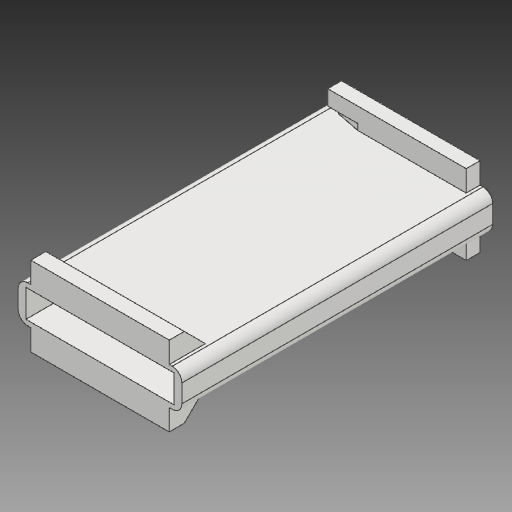
# Autodesk Inventor part: Spulenkoerper
Saved by Autodesk Inventor 2019.4 (Build 234330000, 330)
## iProperties
Part Number: Spulenkoerper
Material: PC/ABS-Kunststoff
Document SubType Name: Modeling
Designer: rYan
Density: 0.357273 g/cm^3
Appearance: Glatt - Weiß
Mass: 1.37233 g
Surface Area: 70.9009 cm^2
Volume: 3.84113 cm^3
Author: rYan
Autodesk Inventor part; units mm, degrees
ref_plane "YZ Plane" through (0, 0, 0) normal (1, 0, 0) x (0, 1, 0)
ref_plane "XZ Plane" through (0, 0, 0) normal (0, 1, 0) x (-1, 0, 0)
ref_plane "XY Plane" through (0, 0, 0) normal (0, 0, 1) x (1, 0, 0)
sketch "Skizze2" plane through (0, 0, 0) normal (0, 1, 0) x (-1, 0, 0)
  line L0 (-12.3, -2.3) -> (12.3, -2.3)
  line L1 (12.3, -2.3) -> (12.3, 2.3)
  line L2 (12.3, 2.3) -> (-12.3, 2.3)
  line L3 (-12.3, 2.3) -> (-12.3, -2.3)
  line L4 (-12.3, -2.3) -> (12.3, 2.3) construction
  line L5 (12.3, -2.3) -> (-12.3, 2.3) construction
  line L6 (-12, 3.1) -> (12, 3.1)
  line L7 (12, -3.1) -> (-12, -3.1)
  line L8 (-19.5039, 0) -> (19.5039, 0) projected
  line L9 (0, -4.8039) -> (0, 4.8039) projected
  arc A0 (-12, 3.1) -> (-13.6, 1.5) centre (-12, 1.5) ccw
  arc A1 (-13.6, -1.5) -> (-12, -3.1) centre (-12, -1.5) ccw
  arc A2 (13.6, 1.5) -> (12, 3.1) centre (12, 1.5) ccw
  arc A3 (12, -3.1) -> (13.6, -1.5) centre (12, -1.5) ccw
  line L10 (-13.6, 1.5) -> (-13.6, -1.5)
  line L11 (13.6, 1.5) -> (13.6, -1.5)
  point P0 (0, 0)
  dimension "d0" = 24.6
  dimension "d1" = 4.6
  dimension "d2" = 0.8
  dimension "d29" = 3.2
  dimension "d32" = 1.3
  constraints: 20 end point, 8 point on circle, 5 tangent, 4 centre point, 4 parallel, 2 midpoint, 1 horizontal, 1 perpendicular, 1 vertical, 4 other
  measures "d0" distance of L2.end L1.end
  measures "d1" distance of L1.end L0.end
  measures "d2" distance between parallel lines of L2 L6
  measures "d29" diameter of A0
  measures "d32" distance between parallel lines of L10 L3
extrude "Extrusion1" add sketch "Skizze2" along normal blind 25.9 contours L0 L9 L7 A1 L10 L8 L3 | L0 L1 L8 L11 A3 L7 L9 | L8 L10 A0 L6 L9 L2 L3 | L1 L2 L9 L6 A2 L11 L8
sketch "Skizze3" plane through (0, 25.9, 0) normal (0, 1, 0) x (1, 0, 0)
  line L0 (12.3, 2.3) -> (12.3, -2.3) projected
  line L1 (12.3, -2.3) -> (-12.3, -2.3) projected
  line L2 (-12.3, -2.3) -> (-12.3, 2.3) projected
  line L3 (-12.3, 2.3) -> (12.3, 2.3) projected
  line L4 (12, 3.1) -> (-12, 3.1) projected
  line L5 (-12, -3.1) -> (12, -3.1) projected
  line L6 (19.0715, 0) -> (-19.0452, 0) projected
  line L7 (11.5, -3.1) -> (-11.5, -3.1)
  line L8 (-11.5, -3.1) -> (-11.5, -6.6)
  line L9 (-11.5, -6.6) -> (11.5, -6.6)
  line L10 (11.5, -6.6) -> (11.5, -3.1)
  line L11 (12, 3.1) -> (-12, 3.1) projected
  line L12 (11.5, 3.1) -> (-11.5, 3.1)
  line L13 (-11.5, 3.1) -> (-11.5, 6.6)
  line L14 (-11.5, 6.6) -> (11.5, 6.6)
  line L15 (11.5, 6.6) -> (11.5, 3.1)
  line L16 (0, 7.84) -> (0, -7.84) projected
  line L17 (-12, -3.1) -> (12, -3.1) projected
  arc A0 (12, -3.1) -> (13.6, -1.5) centre (12, -1.5) ccw projected
  arc A1 (13.6, 1.5) -> (12, 3.1) centre (12, 1.5) ccw projected
  arc A2 (-12, 3.1) -> (-13.6, 1.5) centre (-12, 1.5) ccw projected
  arc A3 (-13.6, -1.5) -> (-12, -3.1) centre (-12, -1.5) ccw projected
  line L18 (13.6, -1.5) -> (13.6, 1.5) projected
  line L19 (-13.6, 1.5) -> (-13.6, -1.5) projected
  dimension "d18" = 3.5
  dimension "d19" = 23
  constraints: 16 end point, 4 parallel, 3 point on line, 2 horizontal, 2 perpendicular, 3 other
  measures "d18" distance of L7.end L8.end
  measures "d19" distance of L8.end L9.end
extrude "Extrusion2" add sketch "Skizze3" against normal blind 2.5 contours L16 L14 L15 L4 | L4 L13 L14 L16 | L16 L9 L8 L5 | L5 L10 L9 L16
mirror "Spiegeln1" about plane through (0, 0, 0) normal (0, 1, 0) of "Extrusion1", "Extrusion2"
chamfer "Fase1" distance 3.5 angle 45 2 edges at (0, -23.4, 3.1) (0, -23.4, -3.1)
sketch "Skizze7" plane through (0, 23.4, 0) normal (0, -1, 0) x (1, 0, 0)
  line L0 (13.4387, -2.2) -> (13.6, -2.2) projected
  line L1 (13.6, 1.5) -> (13.6, 2.2) projected
  line L2 (13.6, 2.2) -> (13.4387, 2.2) projected
  line L3 (11.5, 3.1) -> (11.5, 6.6) projected
  line L4 (11.5, 6.6) -> (-11.5, 6.6) projected
  line L5 (-11.5, 6.6) -> (-11.5, 3.1) projected
  line L6 (11.5, 3.1) -> (-11.5, 3.1) projected
  line L7 (-11.5, -3.1) -> (11.5, -3.1) projected
  line L8 (-11.5, -3.1) -> (-11.5, -6.6) projected
  line L9 (-11.5, -6.6) -> (11.5, -6.6) projected
  line L10 (11.5, -6.6) -> (11.5, -3.1) projected
  line L11 (-13.6, -2.2) -> (-13.4387, -2.2) projected
  line L12 (-13.4387, 2.2) -> (-13.6, 2.2) projected
  line L13 (-13.6, -1.5) -> (-13.6, -2.2) projected
  line L14 (-13.6, 2.2) -> (-13.6, 1.5) projected
  arc A0 (-13.6, -1.5) -> (-13.4387, -2.2) centre (-12, -1.5) ccw projected
  arc A1 (-13.4387, 2.2) -> (-13.6, 1.5) centre (-12, 1.5) ccw projected
  arc A2 (13.4387, -2.2) -> (13.6, -1.5) centre (12, -1.5) ccw projected
  line L15 (13.6, -2.2) -> (13.6, -1.5) projected
  arc A3 (13.6, 1.5) -> (13.4387, 2.2) centre (12, 1.5) ccw projected
extrude "Extrusion4" [suppressed]
chamfer "Fase2" [suppressed]
sketch "Skizze8" plane through (-11.5, 23.4, 3.1) normal (0, 0, 1) x (1, 0, 0)
  line L0 (0, 2.5) -> (23, 2.5) projected
  line L1 (0, 2.5) -> (0, 0) projected
  line L2 (23, 0) -> (0, 0) projected
  line L3 (23, 2.5) -> (23, 0) projected
  line L4 (0, 0) -> (23, 0) projected
  line L5 (0, 0) -> (0, 1)
  line L6 (0, 1) -> (5, 0)
  line L7 (5, 0) -> (0, 0)
  point P0 (11.5, -23.4)
  dimension "d33" = 1
  dimension "d34" = 5
  constraints: 6 end point, 2 point on line, 1 collinear
  measures "d33" distance of L1.end L5.end
  measures "d34" distance of L6.end L1.end
extrude "Extrusion5" cut sketch "Skizze8" along normal blind 1 contours L6 L2 L1
sketch "Skizze9" plane through (-11.5, 25.9, 3.1) normal (-1, 0, 0) x (0, 0, 1)
  line L0 (0, -1.5) -> (1, -1.5) projected
  line L1 (1, -1.5) -> (1, -2.5) projected
  line L2 (3.5, -2.5) -> (1, -2.5) projected
  line L3 (3.5, 0) -> (3.5, -2.5) projected
  line L4 (0, 0) -> (3.5, 0) projected
  line L5 (0, -1.5) -> (0, 0) projected
  line L6 (1, -2.5) -> (0, -2.5)
  line L7 (0, -2.5) -> (0, 0)
  line L8 (0, 0) -> (1, 0)
  line L9 (1, 0) -> (1, -2.5)
  point P0 (-3.1, -25.9)
  constraints: 8 end point, 2 parallel, 1 horizontal, 1 perpendicular
extrude "Extrusion6" cut sketch "Skizze9" against normal blind 1 contours L5 L4 L9 L0 | L0 L1 L6 L7
chamfer "Fase3" distance 0.2 angle 45 16 edges at (0, 25.9, 6.6) (11.5, 25.9, 4.85) (13.1314, 25.9, 2.6314) (13.6, 25.9, 0) (13.1314, 25.9, -2.6314) (11.75, 25.9, -3.1) (11.75, 25.9, 3.1) (11.5, 25.9, -4.85) (0, 25.9, -6.6) (-11.5, 25.9, -4.85) (-11.75, 25.9, -3.1) (-13.1314, 25.9, -2.6314) (-13.6, 25.9, 0) (-13.1314, 25.9, 2.6314) (-11.25, 25.9, 3.1) (-11.5, 25.9, 5.35)
